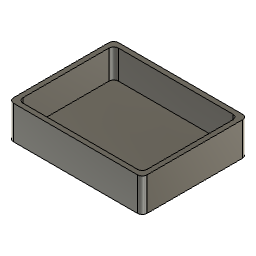
Initial Box Design (Autodesk Fusion 360 design; units mm, degrees)
Autodesk Fusion 360 part; units mm, degrees
sketch "Sketch1" plane through (0, 0, 0) normal (0, 0, 1) x (1, 0, 0) in component "Component"
  line L0 (70, 55) -> (-70, 55)
  line L1 (-70, 55) -> (-70, -55)
  line L2 (-70, -55) -> (70, -55)
  line L3 (70, -55) -> (70, 55)
  line L4 (70, 55) -> (-70, -55) construction
  line L5 (-70, 55) -> (70, -55) construction
  dimension "d1" = 140
  dimension "d2" = 110
  constraint horizontal L0
  constraint perpendicular L0 L1
  constraint parallel L0 L2
  constraint parallel L1 L3
  constraint coincident L4 origin
  constraint coincident L5 origin
  measures "d1" distance of L1.end L2.end
  measures "d2" distance of L0.end L1.end
extrude "Extrude1" add sketch "Sketch1" along normal blind 35 in component "Component"
sketch "Sketch3" plane through (0, 0, 35) normal (0, 0, 1) x (-1, 0, 0) in component "Component"
  line L0 (-70, 55) -> (-70, -55)
  line L1 (-70, -55) -> (70, -55)
  line L2 (70, -55) -> (70, 55)
  line L3 (70, 55) -> (-70, 55)
  line L4 (65, -50) -> (-65, -50)
  line L5 (-65, -50) -> (-65, 50)
  line L6 (-65, 50) -> (65, 50)
  line L7 (65, 50) -> (65, -50)
  line L8 (65, -50) -> (-65, 50) construction
  line L9 (-65, -50) -> (65, 50) construction
  dimension "d5" = 130
  dimension "d6" = 100
  constraint horizontal L4
  constraint perpendicular L4 L5
  constraint parallel L4 L6
  constraint parallel L5 L7
  constraint coincident L8 origin
  constraint coincident L9 origin
  measures "d5" distance of L5.end L6.end
  measures "d6" distance of L4.end L5.end
extrude "Extrude2" cut sketch "Sketch3" against normal up to surface (30 mm away) contours L4 L5 L6 L7 in component "Component"
fillet "Fillet1" radius 5 4 edges at (65, -50, 20) (65, 50, 20) (-65, 50, 20) (-65, -50, 20) in component "Component"
fillet "Fillet2" radius 5 4 edges at (-70, 55, 17.5) (-70, -55, 17.5) (70, -55, 17.5) (70, 55, 17.5) in component "Component"
component "Component" placed x (1, 0, 0) y (0, 1, 0) z (0, 0, 1) at (0, 0, 0)
